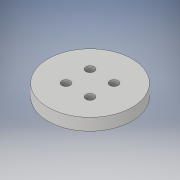
# Autodesk Inventor part: Motor_Testmount
Saved by Autodesk Inventor 2019.4 (Build 234330000, 330)
## iProperties
Created: 2019-10-15
Part Number: Motor_Testmount
Material: Generic
Document SubType Name: Modeling
Designer: Jorian Bruslind
Density: 1 g/cm^3
Appearance: Default
Author: Jorian Bruslind
Autodesk Inventor part; units mm, degrees
ref_plane "YZ Plane" through (0, 0, 0) normal (1, 0, 0) x (0, 1, 0)
ref_plane "XZ Plane" through (0, 0, 0) normal (0, 1, 0) x (-1, 0, 0)
ref_plane "XY Plane" through (0, 0, 0) normal (0, 0, 1) x (1, 0, 0)
sketch "Sketch1" plane through (0, 0, 0) normal (0, 1, 0) x (-1, 0, 0)
  line L0 (0, 0) -> (70, 0) construction
  circle A0 centre (0, 0) radius 17.5
  line L1 (0, 0) -> (0, -5)
  line L2 (0, -5) -> (5, -5)
  circle A1 centre (5, -5) radius 1.75
  circle A2 centre (-5, -5) radius 1.75
  circle A3 centre (5, 5) radius 1.75
  circle A4 centre (-5, 5) radius 1.75
  dimension "d2" = 35
  dimension "d3" = 5
  dimension "d4" = 5
  dimension "d5" = 3.5
  dimension "d8" = 10
  dimension "d11" = 10
  constraints: 6 end point, 5 centre point, 2 coincident, 2 horizontal, 2 vertical, 1 perpendicular, 6 other
  measures "d2" diameter of A0
  measures "d3" distance of L1.start L1.end
  measures "d4" distance of L1.end L2.end
  measures "d5" diameter of A1
  measures "d8" distance of A1.centre A2.centre
  measures "d11" distance of A1.centre A3.centre
extrude "Extrusion1" add sketch "Sketch1" along normal blind 5
body "Solid1"
